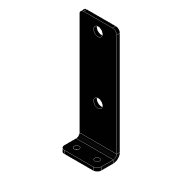
# Autodesk Inventor part: steel_plate7
Saved by Autodesk Inventor 2022 (Build 260153000, 153)
## iProperties
Created: 2021-08-07
Part Number: steel_plate7
Material: 鋼、炭素鋼
Document SubType Name: Sheet Metal
Designer: yuta0
Density: 7.85 g/cm^3
Sheet Metal Rule: Default_mm
Appearance: 滑らか - 黒
Mass: 13.7995 g
Surface Area: 25.202 cm^2
Volume: 1.75789 cm^3
在庫数: 0.0
購入先: Meviy
Author: yuta0
Autodesk Inventor part; units mm, degrees
ref_plane "YZ Plane" through (0, 0, 0) normal (1, 0, 0) x (0, 1, 0)
ref_plane "XZ Plane" through (0, 0, 0) normal (0, 1, 0) x (-1, 0, 0)
ref_plane "XY Plane" through (0, 0, 0) normal (0, 0, 1) x (1, 0, 0)
sketch "スケッチ1" plane through (0, 0, 0) normal (0, 0, 1) x (1, 0, 0)
  line L0 (-9, -27.5) -> (9, -27.5)
  line L1 (9, -27.5) -> (9, 27.5)
  line L2 (9, 27.5) -> (-9, 27.5)
  line L3 (-9, 27.5) -> (-9, -27.5)
  line L4 (-9, -27.5) -> (9, 27.5) construction
  line L5 (9, -27.5) -> (-9, 27.5) construction
  point P0 (0, 0)
  dimension "d0" = 18
  dimension "d1" = 55
  measures "d0" distance of L1.end L2.end
  measures "d1" distance of L0.end L1.end
extrude "プレート1" add sketch "スケッチ1" along normal blind 1.6
sketch "スケッチ2" plane through (9, -25.9, 0) normal (0, -1, 0) x (1, 0, 0)
  line L0 (-18, 0) -> (0, 0)
  line L1 (0, 0) -> (0, 11)
  line L2 (0, 11) -> (-18, 11)
  line L3 (-18, 11) -> (-18, 0)
  constraints: 6 end point, 1 horizontal, 1 perpendicular, 1 vertical
edge flange "フランジ1" height 11 angle 90 thickness 1.6 bend radius 1.6 thickness toward (0, -1, 0) relief tear relief width 1.6 relief depth 0.8 edges at (0, -27.5, 1.6) wall of the first edge with corners at (-9, -25.9, 0) (9, -25.9, 0) (9, -25.9, 11) (-9, -25.9, 11)
bend "曲げ1"
corner "コーナー1"
sketch "スケッチ3" plane through (0, 0, 1.6) normal (0, 0, 1) x (1, 0, 0)
  line L0 (-9, 27.5) -> (9, 27.5) projected
  point P0 (0, 0)
  point P1 (0, 22.5)
  point P2 (0, -7.5)
  dimension "d13" = 5
  dimension "d14" = 30
  constraints: 2 vertical alignment
  measures "d13" distance from line of L0 point (0, 22.5)
  measures "d14" distance of point (0, -7.5) point (0, 22.5)
hole "穴1" at (0, 22.5, 1.6) at (0, -7.5, 1.6) direction (0, 0, -1) diameter 4.3 end through all clearance for "Flat Head Machine Screw" size "M4" standard "Ansi Metric M Profile"
sketch "スケッチ4" plane through (-9, -27.5, 11) normal (0, -1, 0) x (1, 0, 0)
  line L0 (0, 0) -> (18, 0) projected
  line L1 (18, 0) -> (18, -7.8) projected
  line L2 (0, -7.8) -> (0, 0) projected
  point P0 (9, -11)
  point P1 (14, -4)
  point P2 (4, -4)
  dimension "d22" = 4
  dimension "d40" = 4
  dimension "d41" = 4
  constraints: 1 horizontal alignment, 1 other
  measures "d22" distance from line of L0 point (14, -4)
  measures "d41" distance from line of L1 point (14, -4)
hole "穴2" at (5, -27.5, 7) at (-5, -27.5, 7) direction (0, 1, 0) diameter 2.459 end through all thread size "M3x0.5" class "6H" standard "ANSI Metric M Profile"
fillet "コーナーR1" radius 2 3 edges at (9, -26.7, 11) (-9, 27.5, 0.8) (9, 27.5, 0.8)
fillet "コーナーR2" radius 2 1 edges at (-9, -26.7, 11)
equation "\"d20\" = Thickness"
equation "\"d30\" = Thickness"
equation "\"d2\" = Thickness"
equation "\"d3\" = BendReliefWidth"
equation "\"d4\" = BendReliefDepth"
equation "\"d5\" = MinimumRemnant"
equation "\"d6\" = TransitionRadius"
equation "\"d9\" = BendRadius"
equation "\"d10\" = CornerReliefSize"
equation "\"d11\" = GapSize"
equation "\"d12\" = JacobiRadiusSize"
equation "\"BendRadius\" = Thickness"
equation "\"BendReliefWidth\" = Thickness"
equation "\"BendReliefDepth\" = 0.5 * Thickness"
equation "\"CornerReliefSize\" = 4 * Thickness"
equation "\"MinimumRemnant\" = 2 * Thickness"
equation "\"TransitionRadius\" = BendRadius"
equation "\"JacobiRadiusSize\" = BendRadius"
equation "\"GapSize\" = Thickness"
equation "\"Thickness\" = 1.6"
